Autodesk Fusion 360 part; units mm, degrees
note: some values were not read from the file. Set by a fixed rule: which sketch regions a step uses.
(part 36 of 59)
  spline S12 degree 5 poles (-26.8955, 1.5338) (-26.8956, 1.5338) (-26.8958, 1.5337) (-26.8961, 1.5336) (-26.8966, 1.5334) (-26.8973, 1.5331) (-26.8981, 1.5328) (-26.899, 1.5324) (-26.9, 1.5319) (-26.9011, 1.5315) (-26.9023, 1.5309) (-26.9036, 1.5304) (-26.905, 1.5298) (-26.9065, 1.5291) (-26.908, 1.5284) (-26.9097, 1.5276) (-26.9115, 1.5269) (-26.9134, 1.526) (-26.9153, 1.5251) (-26.9173, 1.5242) (-26.9195, 1.5232) (-26.9217, 1.5222) (-26.924, 1.5212) (-26.9263, 1.5201) (-26.9288, 1.5189) (-26.9313, 1.5177) (-26.9339, 1.5165) (-26.9366, 1.5152) (-26.9394, 1.5139) (-26.9423, 1.5125) (-26.9452, 1.5111) (-26.9482, 1.5097) (-26.9513, 1.5082) (-26.9544, 1.5066) (-26.9577, 1.5051) (-26.961, 1.5034) (-26.9643, 1.5018) (-26.9678, 1.5001) (-26.9713, 1.4983) (-26.9748, 1.4965) (-26.9785, 1.4947) (-26.9822, 1.4928) (-26.986, 1.4909) (-26.9898, 1.4889) (-26.9937, 1.4869) (-26.9977, 1.4849) (-27.0017, 1.4828) (-27.0058, 1.4807) (-27.01, 1.4785) (-27.0142, 1.4763) (-27.0185, 1.4741) (-27.0228, 1.4718) (-27.0272, 1.4694) (-27.0317, 1.4671) (-27.0362, 1.4647) (-27.0408, 1.4622) (-27.0454, 1.4597) (-27.0501, 1.4572) (-27.0549, 1.4546) (-27.0597, 1.452) (-27.0645, 1.4493) (-27.0694, 1.4466) (-27.0744, 1.4439) (-27.0794, 1.4411) (-27.0845, 1.4383) (-27.0896, 1.4354) (-27.0948, 1.4325) (-27.1, 1.4296) (-27.1053, 1.4266) (-27.1106, 1.4236) (-27.116, 1.4205) (-27.1214, 1.4174) (-27.1269, 1.4143) (-27.1324, 1.4111) (-27.138, 1.4079) (-27.1436, 1.4046) (-27.1493, 1.4013) (-27.155, 1.398) (-27.1608, 1.3946) (-27.1666, 1.3912) (-27.1725, 1.3877) (-27.1784, 1.3842) (-27.1843, 1.3807) (-27.1903, 1.3771) (-27.1963, 1.3735) (-27.2024, 1.3699) (-27.2085, 1.3662) (-27.2147, 1.3624) (-27.2209, 1.3587) (-27.2271, 1.3549) (-27.2334, 1.351) (-27.2397, 1.3471) (-27.2461, 1.3432) (-27.2525, 1.3392) (-27.259, 1.3352) (-27.2654, 1.3312) (-27.272, 1.3271) (-27.2785, 1.323) (-27.2851, 1.3188) (-27.2918, 1.3146) (-27.2985, 1.3104) (-27.3052, 1.3061) (-27.3119, 1.3018) (-27.3187, 1.2975) (-27.3256, 1.2931) (-27.3324, 1.2887) (-27.3393, 1.2842) (-27.3463, 1.2797) (-27.3533, 1.2752) (-27.3603, 1.2706) (-27.3673, 1.266) (-27.3744, 1.2613) (-27.3815, 1.2566) (-27.3887, 1.2519) (-27.3958, 1.2471) (-27.4031, 1.2423) (-27.4103, 1.2375) (-27.4176, 1.2326) (-27.4249, 1.2277) (-27.4323, 1.2227) (-27.4396, 1.2177) (-27.447, 1.2127) (-27.4545, 1.2076) (-27.462, 1.2025) (-27.4695, 1.1974) (-27.477, 1.1922) (-27.4846, 1.187) (-27.4922, 1.1817) (-27.4998, 1.1765) (-27.5074, 1.1711) (-27.5151, 1.1658) (-27.5228, 1.1604) (-27.5306, 1.1549) (-27.5384, 1.1494) (-27.5462, 1.1439) (-27.554, 1.1384) (-27.5618, 1.1328) (-27.5697, 1.1272) (-27.5776, 1.1215) (-27.5856, 1.1158) (-27.5936, 1.1101) (-27.6015, 1.1043) (-27.6096, 1.0985) (-27.6176, 1.0926) (-27.6257, 1.0868) (-27.6338, 1.0808) (-27.6419, 1.0749) (-27.6501, 1.0689) (-27.6582, 1.0629) (-27.6665, 1.0568) (-27.6747, 1.0507) (-27.6829, 1.0446) (-27.6912, 1.0384) (-27.6995, 1.0322) (-27.7078, 1.0259) (-27.7162, 1.0197) (-27.7246, 1.0133) (-27.733, 1.007) (-27.7414, 1.0006) (-27.7498, 0.9942) (-27.7583, 0.9877) (-27.7668, 0.9812) (-27.7753, 0.9747) (-27.7838, 0.9681) (-27.7924, 0.9615) (-27.801, 0.9548) (-27.8096, 0.9482) (-27.8182, 0.9415) (-27.8268, 0.9347) (-27.8355, 0.9279) (-27.8442, 0.9211) (-27.8529, 0.9142) (-27.8616, 0.9073) (-27.8704, 0.9004) (-27.8791, 0.8935) (-27.8879, 0.8865) (-27.8967, 0.8794) (-27.9055, 0.8724) (-27.9144, 0.8652) (-27.9233, 0.8581) (-27.9322, 0.8509) (-27.9411, 0.8437) (-27.95, 0.8365) (-27.9589, 0.8292) (-27.9679, 0.8219) (-27.9769, 0.8145) (-27.9859, 0.8071) (-27.9949, 0.7997) (-28.0039, 0.7922) (-28.013, 0.7847) (-28.0221, 0.7772) (-28.0312, 0.7697) (-28.0403, 0.7621) (-28.0494, 0.7544) (-28.0585, 0.7468) (-28.0677, 0.7391) (-28.0769, 0.7313) (-28.0861, 0.7235) (-28.0953, 0.7157) (-28.1045, 0.7079) (-28.1137, 0.7) (-28.123, 0.6921) (-28.1323, 0.6842) (-28.1416, 0.6762) (-28.1509, 0.6682) (-28.1602, 0.6601) (-28.1695, 0.652) (-28.1789, 0.6439) (-28.1882, 0.6357) (-28.1976, 0.6276) (-28.207, 0.6193) (-28.2164, 0.6111) (-28.2259, 0.6028) (-28.2353, 0.5945) (-28.2447, 0.5861) (-28.2542, 0.5777) (-28.2637, 0.5693) (-28.2732, 0.5608) (-28.2827, 0.5523) (-28.2922, 0.5438) (-28.3018, 0.5352) (-28.3113, 0.5266) (-28.3209, 0.518) (-28.3305, 0.5093) (-28.34, 0.5006) (-28.3496, 0.4919) (-28.3593, 0.4831) (-28.3689, 0.4743) (-28.3785, 0.4655) (-28.3882, 0.4566) (-28.3978, 0.4477) (-28.4075, 0.4387) (-28.4172, 0.4298) (-28.4269, 0.4208) (-28.4366, 0.4117) (-28.4464, 0.4027) (-28.4561, 0.3935) (-28.4658, 0.3844) (-28.4756, 0.3752) (-28.4854, 0.366) (-28.4951, 0.3568) (-28.503, 0.3494) (-28.5089, 0.3438) (-28.5128, 0.34) (-28.5147, 0.3382) knots 0 0 0 0 0 0 0.00416667 0.00833333 0.0125 0.01666667 0.02083333 0.025 0.02916667 0.03333333 0.0375 0.04166667 0.04583333 0.05 0.05416667 0.05833333 0.0625 0.06666667 0.07083333 0.075 0.07916667 0.08333333 0.0875 0.09166667 0.09583333 0.1 0.10416667 0.10833333 0.1125 0.11666667 0.12083333 0.125 0.12916667 0.13333333 0.1375 0.14166667 0.14583333 0.15 0.15416667 0.15833333 0.1625 0.16666667 0.17083333 0.175 0.17916667 0.18333333 0.1875 0.19166667 0.19583333 0.2 0.20416667 0.20833333 0.2125 0.21666667 0.22083333 0.225 0.22916667 0.23333333 0.2375 0.24166667 0.24583333 0.25 0.25416667 0.25833333 0.2625 0.26666667 0.27083333 0.275 0.27916667 0.28333333 0.2875 0.29166667 0.29583333 0.3 0.30416667 0.30833333 0.3125 0.31666667 0.32083333 0.325 0.32916667 0.33333333 0.3375 0.34166667 0.34583333 0.35 0.35416667 0.35833333 0.3625 0.36666667 0.37083333 0.375 0.37916667 0.38333333 0.3875 0.39166667 0.39583333 0.4 0.40416667 0.40833333 0.4125 0.41666667 0.42083333 0.425 0.42916667 0.43333333 0.4375 0.44166667 0.44583333 0.45 0.45416667 0.45833333 0.4625 0.46666667 0.47083333 0.475 0.47916667 0.48333333 0.4875 0.49166667 0.49583333 0.5 0.50416667 0.50833333 0.5125 0.51666667 0.52083333 0.525 0.52916667 0.53333333 0.5375 0.54166667 0.54583333 0.55 0.55416667 0.55833333 0.5625 0.56666667 0.57083333 0.575 0.57916667 0.58333333 0.5875 0.59166667 0.59583333 0.6 0.60416667 0.60833333 0.6125 0.61666667 0.62083333 0.625 0.62916667 0.63333333 0.6375 0.64166667 0.64583333 0.65 0.65416667 0.65833333 0.6625 0.66666667 0.67083333 0.675 0.67916667 0.68333333 0.6875 0.69166667 0.69583333 0.7 0.70416667 0.70833333 0.7125 0.71666667 0.72083333 0.725 0.72916667 0.73333333 0.7375 0.74166667 0.74583333 0.75 0.75416667 0.75833333 0.7625 0.76666667 0.77083333 0.775 0.77916667 0.78333333 0.7875 0.79166667 0.79583333 0.8 0.80416667 0.80833333 0.8125 0.81666667 0.82083333 0.825 0.82916667 0.83333333 0.8375 0.84166667 0.84583333 0.85 0.85416667 0.85833333 0.8625 0.86666667 0.87083333 0.875 0.87916667 0.88333333 0.8875 0.89166667 0.89583333 0.9 0.90416667 0.90833333 0.9125 0.91666667 0.92083333 0.925 0.92916667 0.93333333 0.9375 0.94166667 0.94583333 0.95 0.95416667 0.95833333 0.9625 0.96666667 0.97083333 0.975 0.97916667 0.98333333 0.9875 0.99166667 0.99583333 1 1 1 1 1 1
  arc A13 (-28.5147, 0.3382) -> (-28.1181, -0.5527) centre (0, 12.5) ccw
  spline S13 degree 5 poles (-28.1181, -0.5527) (-28.1154, -0.5525) (-28.11, -0.5521) (-28.1019, -0.5515) (-28.0911, -0.5506) (-28.0777, -0.5495) (-28.0644, -0.5484) (-28.051, -0.5473) (-28.0377, -0.5462) (-28.0244, -0.5451) (-28.0112, -0.5439) (-27.9979, -0.5427) (-27.9848, -0.5415) (-27.9716, -0.5404) (-27.9585, -0.5391) (-27.9454, -0.5379) (-27.9323, -0.5367) (-27.9193, -0.5354) (-27.9063, -0.5342) (-27.8934, -0.5329) (-27.8805, -0.5316) (-27.8676, -0.5303) (-27.8547, -0.529) (-27.8419, -0.5276) (-27.8291, -0.5263) (-27.8164, -0.5249) (-27.8037, -0.5236) (-27.791, -0.5222) (-27.7784, -0.5208) (-27.7658, -0.5194) (-27.7532, -0.518) (-27.7406, -0.5165) (-27.7281, -0.5151) (-27.7157, -0.5136) (-27.7032, -0.5122) (-27.6908, -0.5107) (-27.6785, -0.5092) (-27.6661, -0.5077) (-27.6539, -0.5062) (-27.6416, -0.5047) (-27.6294, -0.5031) (-27.6172, -0.5016) (-27.605, -0.5) (-27.5929, -0.4984) (-27.5809, -0.4968) (-27.5688, -0.4952) (-27.5568, -0.4936) (-27.5449, -0.492) (-27.5329, -0.4904) (-27.521, -0.4887) (-27.5092, -0.4871) (-27.4974, -0.4854) (-27.4856, -0.4838) (-27.4738, -0.4821) (-27.4621, -0.4804) (-27.4505, -0.4787) (-27.4388, -0.477) (-27.4273, -0.4752) (-27.4157, -0.4735) (-27.4042, -0.4718) (-27.3927, -0.47) (-27.3813, -0.4682) (-27.3699, -0.4665) (-27.3585, -0.4647) (-27.3472, -0.4629) (-27.3359, -0.4611) (-27.3247, -0.4593) (-27.3135, -0.4574) (-27.3023, -0.4556) (-27.2912, -0.4538) (-27.2801, -0.4519) (-27.2691, -0.4501) (-27.2581, -0.4482) (-27.2471, -0.4463) (-27.2362, -0.4445) (-27.2253, -0.4426) (-27.2145, -0.4407) (-27.2037, -0.4388) (-27.1929, -0.4368) (-27.1822, -0.4349) (-27.1715, -0.433) (-27.1609, -0.4311) (-27.1503, -0.4291) (-27.1397, -0.4272) (-27.1292, -0.4252) (-27.1188, -0.4232) (-27.1083, -0.4213) (-27.0979, -0.4193) (-27.0876, -0.4173) (-27.0773, -0.4153) (-27.0671, -0.4133) (-27.0568, -0.4113) (-27.0467, -0.4093) (-27.0365, -0.4072) (-27.0265, -0.4052) (-27.0164, -0.4032) (-27.0064, -0.4011) (-26.9965, -0.3991) (-26.9866, -0.3971) (-26.9767, -0.395) (-26.9669, -0.3929) (-26.9571, -0.3909) (-26.9474, -0.3888) (-26.9377, -0.3867) (-26.9281, -0.3847) (-26.9185, -0.3826) (-26.9089, -0.3805) (-26.8994, -0.3784) (-26.89, -0.3763) (-26.8806, -0.3742) (-26.8712, -0.3721) (-26.8619, -0.37) (-26.8526, -0.3679) (-26.8434, -0.3658) (-26.8342, -0.3636) (-26.8251, -0.3615) (-26.816, -0.3594) (-26.8069, -0.3573) (-26.798, -0.3551) (-26.789, -0.353) (-26.7801, -0.3509) (-26.7713, -0.3487) (-26.7625, -0.3466) (-26.7537, -0.3445) (-26.7451, -0.3423) (-26.7364, -0.3402) (-26.7278, -0.338) (-26.7193, -0.3359) (-26.7108, -0.3337) (-26.7023, -0.3316) (-26.6939, -0.3294) (-26.6856, -0.3273) (-26.6773, -0.3251) (-26.669, -0.323) (-26.6608, -0.3208) (-26.6527, -0.3187) (-26.6446, -0.3166) (-26.6365, -0.3144) (-26.6286, -0.3123) (-26.6206, -0.3101) (-26.6127, -0.308) (-26.6049, -0.3058) (-26.5971, -0.3037) (-26.5894, -0.3016) (-26.5817, -0.2994) (-26.5741, -0.2973) (-26.5665, -0.2952) (-26.559, -0.293) (-26.5516, -0.2909) (-26.5442, -0.2888) (-26.5368, -0.2867) (-26.5296, -0.2845) (-26.5223, -0.2824) (-26.5151, -0.2803) (-26.508, -0.2782) (-26.5009, -0.2761) (-26.4939, -0.274) (-26.487, -0.272) (-26.4801, -0.2699) (-26.4733, -0.2678) (-26.4665, -0.2657) (-26.4598, -0.2637) (-26.4531, -0.2616) (-26.4465, -0.2596) (-26.4399, -0.2575) (-26.4335, -0.2555) (-26.427, -0.2534) (-26.4207, -0.2514) (-26.4144, -0.2494) (-26.4081, -0.2474) (-26.4019, -0.2454) (-26.3958, -0.2434) (-26.3897, -0.2414) (-26.3837, -0.2395) (-26.3778, -0.2375) (-26.3719, -0.2356) (-26.3661, -0.2336) (-26.3604, -0.2317) (-26.3547, -0.2298) (-26.3491, -0.2279) (-26.3435, -0.226) (-26.338, -0.2241) (-26.3326, -0.2222) (-26.3273, -0.2204) (-26.322, -0.2185) (-26.3167, -0.2167) (-26.3116, -0.2149) (-26.3065, -0.2131) (-26.3015, -0.2113) (-26.2965, -0.2095) (-26.2916, -0.2077) (-26.2868, -0.206) (-26.282, -0.2043) (-26.2774, -0.2026) (-26.2728, -0.2009) (-26.2682, -0.1992) (-26.2638, -0.1975) (-26.2594, -0.1959) (-26.255, -0.1943) (-26.2508, -0.1927) (-26.2466, -0.1911) (-26.2425, -0.1895) (-26.2385, -0.188) (-26.2345, -0.1864) (-26.2307, -0.1849) (-26.2269, -0.1834) (-26.2231, -0.182) (-26.2195, -0.1806) (-26.2159, -0.1791) (-26.2124, -0.1778) (-26.209, -0.1764) (-26.2057, -0.175) (-26.2024, -0.1737) (-26.1993, -0.1724) (-26.1962, -0.1712) (-26.1932, -0.1699) (-26.1903, -0.1687) (-26.1874, -0.1676) (-26.1847, -0.1664) (-26.182, -0.1653) (-26.1794, -0.1642) (-26.1769, -0.1631) (-26.1745, -0.1621) (-26.1722, -0.1611) (-26.17, -0.1602) (-26.1678, -0.1592) (-26.1658, -0.1583) (-26.1638, -0.1575) (-26.1619, -0.1567) (-26.1602, -0.1559) (-26.1585, -0.1551) (-26.1569, -0.1544) (-26.1554, -0.1538) (-26.154, -0.1531) (-26.1527, -0.1526) (-26.1515, -0.152) (-26.1504, -0.1515) (-26.1495, -0.151) (-26.1486, -0.1506) (-26.1478, -0.1503) (-26.1471, -0.15) (-26.1467, -0.1497) (-26.1464, -0.1496) (-26.1462, -0.1495) (-26.1461, -0.1495) knots -1 -1 -1 -1 -1 -1 -0.99583333 -0.99166667 -0.9875 -0.98333333 -0.97916667 -0.975 -0.97083333 -0.96666667 -0.9625 -0.95833333 -0.95416667 -0.95 -0.94583333 -0.94166667 -0.9375 -0.93333333 -0.92916667 -0.925 -0.92083333 -0.91666667 -0.9125 -0.90833333 -0.90416667 -0.9 -0.89583333 -0.89166667 -0.8875 -0.88333333 -0.87916667 -0.875 -0.87083333 -0.86666667 -0.8625 -0.85833333 -0.85416667 -0.85 -0.84583333 -0.84166667 -0.8375 -0.83333333 -0.82916667 -0.825 -0.82083333 -0.81666667 -0.8125 -0.80833333 -0.80416667 -0.8 -0.79583333 -0.79166667 -0.7875 -0.78333333 -0.77916667 -0.775 -0.77083333 -0.76666667 -0.7625 -0.75833333 -0.75416667 -0.75 -0.74583333 -0.74166667 -0.7375 -0.73333333 -0.72916667 -0.725 -0.72083333 -0.71666667 -0.7125 -0.70833333 -0.70416667 -0.7 -0.69583333 -0.69166667 -0.6875 -0.68333333 -0.67916667 -0.675 -0.67083333 -0.66666667 -0.6625 -0.65833333 -0.65416667 -0.65 -0.64583333 -0.64166667 -0.6375 -0.63333333 -0.62916667 -0.625 -0.62083333 -0.61666667 -0.6125 -0.60833333 -0.60416667 -0.6 -0.59583333 -0.59166667 -0.5875 -0.58333333 -0.57916667 -0.575 -0.57083333 -0.56666667 -0.5625 -0.55833333 -0.55416667 -0.55 -0.54583333 -0.54166667 -0.5375 -0.53333333 -0.52916667 -0.525 -0.52083333 -0.51666667 -0.5125 -0.50833333 -0.50416667 -0.5 -0.49583333 -0.49166667 -0.4875 -0.48333333 -0.47916667 -0.475 -0.47083333 -0.46666667 -0.4625 -0.45833333 -0.45416667 -0.45 -0.44583333 -0.44166667 -0.4375 -0.43333333 -0.42916667 -0.425 -0.42083333 -0.41666667 -0.4125 -0.40833333 -0.40416667 -0.4 -0.39583333 -0.39166667 -0.3875 -0.38333333 -0.37916667 -0.375 -0.37083333 -0.36666667 -0.3625 -0.35833333 -0.35416667 -0.35 -0.34583333 -0.34166667 -0.3375 -0.33333333 -0.32916667 -0.325 -0.32083333 -0.31666667 -0.3125 -0.30833333 -0.30416667 -0.3 -0.29583333 -0.29166667 -0.2875 -0.28333333 -0.27916667 -0.275 -0.27083333 -0.26666667 -0.2625 -0.25833333 -0.25416667 -0.25 -0.24583333 -0.24166667 -0.2375 -0.23333333 -0.22916667 -0.225 -0.22083333 -0.21666667 -0.2125 -0.20833333 -0.20416667 -0.2 -0.19583333 -0.19166667 -0.1875 -0.18333333 -0.17916667 -0.175 -0.17083333 -0.16666667 -0.1625 -0.15833333 -0.15416667 -0.15 -0.14583333 -0.14166667 -0.1375 -0.13333333 -0.12916667 -0.125 -0.12083333 -0.11666667 -0.1125 -0.10833333 -0.10416667 -0.1 -0.09583333 -0.09166667 -0.0875 -0.08333333 -0.07916667 -0.075 -0.07083333 -0.06666667 -0.0625 -0.05833333 -0.05416667 -0.05 -0.04583333 -0.04166667 -0.0375 -0.03333333 -0.02916667 -0.025 -0.02083333 -0.01666667 -0.0125 -0.00833333 -0.00416667 0 0 0 0 0 0
  line L35 (-26.1461, -0.1495) -> (-26.1453, -0.1491)
  line L36 (-26.1453, -0.1491) -> (-25.8803, -0.0209)
  arc A14 (-25.8803, -0.0209) -> (-25.3417, -1.078) centre (0, 12.5) ccw
  line L37 (-25.3417, -1.078) -> (-25.6012, -1.2171)
  line L38 (-25.6012, -1.2171) -> (-25.6019, -1.2175)
  spline S14 degree 5 poles (-25.6019, -1.2175) (-25.602, -1.2175) (-25.6022, -1.2176) (-25.6025, -1.2178) (-25.6029, -1.218) (-25.6036, -1.2184) (-25.6043, -1.2188) (-25.6052, -1.2193) (-25.6061, -1.2198) (-25.6072, -1.2204) (-25.6083, -1.221) (-25.6096, -1.2217) (-25.6109, -1.2225) (-25.6123, -1.2233) (-25.6138, -1.2242) (-25.6154, -1.2251) (-25.6171, -1.2261) (-25.6188, -1.2271) (-25.6207, -1.2282) (-25.6226, -1.2293) (-25.6246, -1.2305) (-25.6267, -1.2317) (-25.6289, -1.233) (-25.6311, -1.2344) (-25.6334, -1.2358) (-25.6358, -1.2372) (-25.6383, -1.2387) (-25.6409, -1.2403) (-25.6435, -1.2419) (-25.6462, -1.2435) (-25.6489, -1.2452) (-25.6518, -1.247) (-25.6547, -1.2488) (-25.6577, -1.2506) (-25.6607, -1.2526) (-25.6638, -1.2545) (-25.667, -1.2565) (-25.6702, -1.2586) (-25.6735, -1.2607) (-25.6769, -1.2628) (-25.6803, -1.265) (-25.6838, -1.2673) (-25.6874, -1.2696) (-25.691, -1.2719) (-25.6947, -1.2743) (-25.6984, -1.2768) (-25.7022, -1.2793) (-25.706, -1.2818) (-25.71, -1.2844) (-25.7139, -1.287) (-25.718, -1.2897) (-25.722, -1.2925) (-25.7262, -1.2952) (-25.7304, -1.2981) (-25.7346, -1.3009) (-25.7389, -1.3039) (-25.7432, -1.3068) (-25.7476, -1.3098) (-25.7521, -1.3129) (-25.7566, -1.316) (-25.7612, -1.3192) (-25.7658, -1.3224) (-25.7704, -1.3256) (-25.7751, -1.3289) (-25.7799, -1.3322) (-25.7847, -1.3356) (-25.7895, -1.339) (-25.7944, -1.3425) (-25.7993, -1.346) (-25.8043, -1.3496) (-25.8093, -1.3532) (-25.8144, -1.3568) (-25.8195, -1.3605) (-25.8247, -1.3643) (-25.8299, -1.3681) (-25.8352, -1.3719) (-25.8405, -1.3758) (-25.8458, -1.3797) (-25.8512, -1.3836) (-25.8566, -1.3876) (-25.8621, -1.3917) (-25.8676, -1.3958) (-25.8731, -1.3999) (-25.8787, -1.4041) (-25.8843, -1.4083) (-25.89, -1.4126) (-25.8957, -1.4169) (-25.9014, -1.4213) (-25.9072, -1.4257) (-25.913, -1.4301) (-25.9188, -1.4346) (-25.9247, -1.4391) (-25.9306, -1.4437) (-25.9366, -1.4483) (-25.9426, -1.4529) (-25.9486, -1.4576) (-25.9547, -1.4624) (-25.9608, -1.4672) (-25.9669, -1.472) (-25.9731, -1.4769) (-25.9793, -1.4818) (-25.9855, -1.4867) (-25.9918, -1.4917) (-25.9981, -1.4967) (-26.0044, -1.5018) (-26.0108, -1.5069) (-26.0172, -1.5121) (-26.0236, -1.5173) (-26.0301, -1.5225) (-26.0366, -1.5278) (-26.0431, -1.5332) (-26.0497, -1.5385) (-26.0563, -1.5439) (-26.0629, -1.5494) (-26.0695, -1.5549) (-26.0762, -1.5604) (-26.0829, -1.566) (-26.0896, -1.5716) (-26.0964, -1.5772) (-26.1032, -1.5829) (-26.11, -1.5887) (-26.1168, -1.5945) (-26.1237, -1.6003) (-26.1306, -1.6061) (-26.1375, -1.612) (-26.1445, -1.618) (-26.1515, -1.6239) (-26.1585, -1.63) (-26.1655, -1.636) (-26.1726, -1.6421) (-26.1796, -1.6483) (-26.1868, -1.6544) (-26.1939, -1.6607) (-26.201, -1.6669) (-26.2082, -1.6732) (-26.2154, -1.6796) (-26.2227, -1.6859) (-26.2299, -1.6924) (-26.2372, -1.6988) (-26.2445, -1.7053) (-26.2518, -1.7119) (-26.2592, -1.7184) (-26.2665, -1.725) (-26.2739, -1.7317) (-26.2813, -1.7384) (-26.2888, -1.7451) (-26.2962, -1.7519) (-26.3037, -1.7587) (-26.3112, -1.7656) (-26.3188, -1.7724) (-26.3263, -1.7794) (-26.3339, -1.7863) (-26.3414, -1.7933) (-26.3491, -1.8004) (-26.3567, -1.8075) (-26.3643, -1.8146) (-26.372, -1.8217) (-26.3797, -1.8289) (-26.3874, -1.8362) (-26.3951, -1.8435) (-26.4029, -1.8508) (-26.4106, -1.8581) (-26.4184, -1.8655) (-26.4262, -1.8729) (-26.434, -1.8804) (-26.4419, -1.8879) (-26.4497, -1.8954) (-26.4576, -1.903) (-26.4655, -1.9106) (-26.4734, -1.9183) (-26.4813, -1.926) (-26.4893, -1.9337) (-26.4972, -1.9415) (-26.5052, -1.9493) (-26.5132, -1.9571) (-26.5212, -1.965) (-26.5292, -1.9729) (-26.5373, -1.9809) (-26.5453, -1.9889) (-26.5534, -1.9969) (-26.5615, -2.005) (-26.5696, -2.0131) (-26.5777, -2.0212) (-26.5858, -2.0294) (-26.594, -2.0376) (-26.6022, -2.0459) (-26.6103, -2.0541) (-26.6185, -2.0625) (-26.6267, -2.0708) (-26.635, -2.0792) (-26.6432, -2.0877) (-26.6514, -2.0961) (-26.6597, -2.1046) (-26.668, -2.1132) (-26.6763, -2.1218) (-26.6846, -2.1304) (-26.6929, -2.139) (-26.7012, -2.1477) (-26.7096, -2.1565) (-26.7179, -2.1652) (-26.7263, -2.174) (-26.7347, -2.1829) (-26.7431, -2.1917) (-26.7515, -2.2006) (-26.7599, -2.2096) (-26.7683, -2.2186) (-26.7767, -2.2276) (-26.7852, -2.2366) (-26.7937, -2.2457) (-26.8021, -2.2549) (-26.8106, -2.264) (-26.8191, -2.2732) (-26.8276, -2.2824) (-26.8361, -2.2917) (-26.8447, -2.301) (-26.8532, -2.3104) (-26.8618, -2.3197) (-26.8703, -2.3291) (-26.8789, -2.3386) (-26.8875, -2.3481) (-26.8961, -2.3576) (-26.9047, -2.3671) (-26.9133, -2.3767) (-26.9219, -2.3863) (-26.9305, -2.396) (-26.9392, -2.4057) (-26.9478, -2.4154) (-26.9565, -2.4252) (-26.9651, -2.435) (-26.9738, -2.4448) (-26.9825, -2.4547) (-26.9912, -2.4646) (-26.9999, -2.4745) (-27.0086, -2.4845) (-27.0173, -2.4945) (-27.026, -2.5045) (-27.0347, -2.5146) (-27.0435, -2.5247) (-27.0522, -2.5349) (-27.061, -2.545) (-27.0697, -2.5553) (-27.0767, -2.5635) (-27.082, -2.5696) (-27.0855, -2.5737) (-27.0873, -2.5758) knots 0 0 0 0 0 0 0.00416667 0.00833333 0.0125 0.01666667 0.02083333 0.025 0.02916667 0.03333333 0.0375 0.04166667 0.04583333 0.05 0.05416667 0.05833333 0.0625 0.06666667 0.07083333 0.075 0.07916667 0.08333333 0.0875 0.09166667 0.09583333 0.1 0.10416667 0.10833333 0.1125 0.11666667 0.12083333 0.125 0.12916667 0.13333333 0.1375 0.14166667 0.14583333 0.15 0.15416667 0.15833333 0.1625 0.16666667 0.17083333 0.175 0.17916667 0.18333333 0.1875 0.19166667 0.19583333 0.2 0.20416667 0.20833333 0.2125 0.21666667 0.22083333 0.225 0.22916667 0.23333333 0.2375 0.24166667 0.24583333 0.25 0.25416667 0.25833333 0.2625 0.26666667 0.27083333 0.275 0.27916667 0.28333333 0.2875 0.29166667 0.29583333 0.3 0.30416667 0.30833333 0.3125 0.31666667 0.32083333 0.325 0.32916667 0.33333333 0.3375 0.34166667 0.34583333 0.35 0.35416667 0.35833333 0.3625 0.36666667 0.37083333 0.375 0.37916667 0.38333333 0.3875 0.39166667 0.39583333 0.4 0.40416667 0.40833333 0.4125 0.41666667 0.42083333 0.425 0.42916667 0.43333333 0.4375 0.44166667 0.44583333 0.45 0.45416667 0.45833333 0.4625 0.46666667 0.47083333 0.475 0.47916667 0.48333333 0.4875 0.49166667 0.49583333 0.5 0.50416667 0.50833333 0.5125 0.51666667 0.52083333 0.525 0.52916667 0.53333333 0.5375 0.54166667 0.54583333 0.55 0.55416667 0.55833333 0.5625 0.56666667 0.57083333 0.575 0.57916667 0.58333333 0.5875 0.59166667 0.59583333 0.6 0.60416667 0.60833333 0.6125 0.61666667 0.62083333 0.625 0.62916667 0.63333333 0.6375 0.64166667 0.64583333 0.65 0.65416667 0.65833333 0.6625 0.66666667 0.67083333 0.675 0.67916667 0.68333333 0.6875 0.69166667 0.69583333 0.7 0.70416667 0.70833333 0.7125 0.71666667 0.72083333 0.725 0.72916667 0.73333333 0.7375 0.74166667 0.74583333 0.75 0.75416667 0.75833333 0.7625 0.76666667 0.77083333 0.775 0.77916667 0.78333333 0.7875 0.79166667 0.79583333 0.8 0.80416667 0.80833333 0.8125 0.81666667 0.82083333 0.825 0.82916667 0.83333333 0.8375 0.84166667 0.84583333 0.85 0.85416667 0.85833333 0.8625 0.86666667 0.87083333 0.875 0.87916667 0.88333333 0.8875 0.89166667 0.89583333 0.9 0.90416667 0.90833333 0.9125 0.91666667 0.92083333 0.925 0.92916667 0.93333333 0.9375 0.94166667 0.94583333 0.95 0.95416667 0.95833333 0.9625 0.96666667 0.97083333 0.975 0.97916667 0.98333333 0.9875 0.99166667 0.99583333 1 1 1 1 1 1
  arc A15 (-27.0873, -2.5758) -> (-26.5997, -3.4204) centre (0, 12.5) ccw
  spline S15 degree 5 poles (-26.5997, -3.4204) (-26.597, -3.4199) (-26.5917, -3.4189) (-26.5837, -3.4174) (-26.5731, -3.4154) (-26.5599, -3.413) (-26.5467, -3.4105) (-26.5335, -3.408) (-26.5204, -3.4055) (-26.5073, -3.4029) (-26.4943, -3.4004) (-26.4812, -3.3979) (-26.4682, -3.3953) (-26.4553, -3.3927) (-26.4424, -3.3902) (-26.4295, -3.3876) (-26.4166, -3.385) (-26.4038, -3.3824) (-26.391, -3.3798) (-26.3783, -3.3771) (-26.3656, -3.3745) (-26.3529, -3.3719) (-26.3403, -3.3692) (-26.3276, -3.3666) (-26.3151, -3.3639) (-26.3025, -3.3612) (-26.29, -3.3585) (-26.2776, -3.3558) (-26.2651, -3.3531) (-26.2528, -3.3504) (-26.2404, -3.3477) (-26.2281, -3.3449) (-26.2158, -3.3422) (-26.2035, -3.3394) (-26.1913, -3.3367) (-26.1792, -3.3339) (-26.167, -3.3311) (-26.1549, -3.3283) (-26.1428, -3.3255) (-26.1308, -3.3227) (-26.1188, -3.3199) (-26.1069, -3.3171) (-26.095, -3.3143) (-26.0831, -3.3115) (-26.0712, -3.3086) (-26.0594, -3.3058) (-26.0477, -3.3029) (-26.0359, -3.3001) (-26.0242, -3.2972) (-26.0126, -3.2943) (-26.001, -3.2914) (-25.9894, -3.2886) (-25.9778, -3.2857) (-25.9663, -3.2828) (-25.9549, -3.2798) (-25.9435, -3.2769) (-25.9321, -3.274) (-25.9207, -3.2711) (-25.9094, -3.2682) (-25.8982, -3.2652) (-25.8869, -3.2623) (-25.8757, -3.2593) (-25.8646, -3.2564) (-25.8535, -3.2534) (-25.8424, -3.2504) (-25.8314, -3.2475) (-25.8204, -3.2445) (-25.8094, -3.2415) (-25.7985, -3.2385) (-25.7877, -3.2355) (-25.7768, -3.2325) (-25.766, -3.2295) (-25.7553, -3.2265) (-25.7446, -3.2235) (-25.7339, -3.2205) (-25.7233, -3.2175) (-25.7127, -3.2145) (-25.7022, -3.2114) (-25.6917, -3.2084) (-25.6812, -3.2054) (-25.6708, -3.2023) (-25.6604, -3.1993) (-25.6501, -3.1963) (-25.6398, -3.1932) (-25.6296, -3.1902) (-25.6194, -3.1871) (-25.6092, -3.1841) (-25.5991, -3.181) (-25.589, -3.1779) (-25.579, -3.1749) (-25.569, -3.1718) (-25.559, -3.1688) (-25.5491, -3.1657) (-25.5393, -3.1626) (-25.5294, -3.1596) (-25.5197, -3.1565) (-25.5099, -3.1534) (-25.5003, -3.1503) (-25.4906, -3.1473) (-25.481, -3.1442) (-25.4715, -3.1411) (-25.462, -3.138) (-25.4525, -3.135) (-25.4431, -3.1319) (-25.4337, -3.1288) (-25.4244, -3.1257) (-25.4151, -3.1227) (-25.4059, -3.1196) (-25.3967, -3.1165) (-25.3876, -3.1134) (-25.3785, -3.1104) (-25.3694, -3.1073) (-25.3604, -3.1042) (-25.3515, -3.1012) (-25.3426, -3.0981) (-25.3337, -3.095) (-25.3249, -3.092) (-25.3161, -3.0889) (-25.3074, -3.0859) (-25.2988, -3.0828) (-25.2901, -3.0798) (-25.2816, -3.0767) (-25.2731, -3.0737) (-25.2646, -3.0706) (-25.2562, -3.0676) (-25.2478, -3.0645) (-25.2394, -3.0615) (-25.2312, -3.0585) (-25.2229, -3.0555) (-25.2148, -3.0524) (-25.2066, -3.0494) (-25.1986, -3.0464) (-25.1905, -3.0434) (-25.1826, -3.0404) (-25.1746, -3.0374) (-25.1668, -3.0344) (-25.1589, -3.0315) (-25.1512, -3.0285) (-25.1434, -3.0255) (-25.1358, -3.0226) (-25.1282, -3.0196) (-25.1206, -3.0166) (-25.1131, -3.0137) (-25.1056, -3.0108) (-25.0982, -3.0078) (-25.0909, -3.0049) (-25.0836, -3.002) (-25.0763, -2.9991) (-25.0691, -2.9962) (-25.062, -2.9933) (-25.0549, -2.9905) (-25.0479, -2.9876) (-25.0409, -2.9848) (-25.034, -2.9819) (-25.0271, -2.9791) (-25.0203, -2.9762) (-25.0136, -2.9734) (-25.0069, -2.9706) (-25.0002, -2.9678) (-24.9936, -2.9651) (-24.9871, -2.9623) (-24.9806, -2.9595) (-24.9742, -2.9568) (-24.9679, -2.9541) (-24.9616, -2.9514) (-24.9553, -2.9486) (-24.9492, -2.946) (-24.943, -2.9433) (-24.937, -2.9406) (-24.931, -2.938) (-24.925, -2.9353) (-24.9192, -2.9327) (-24.9133, -2.9301) (-24.9076, -2.9275) (-24.9019, -2.925) (-24.8962, -2.9224) (-24.8907, -2.9199) (-24.8852, -2.9174) (-24.8797, -2.9149) (-24.8743, -2.9124) (-24.869, -2.9099) (-24.8637, -2.9075) (-24.8585, -2.905) (-24.8534, -2.9026) (-24.8483, -2.9002) (-24.8433, -2.8979) (-24.8384, -2.8955) (-24.8335, -2.8932) (-24.8287, -2.8909) (-24.8239, -2.8886) (-24.8193, -2.8863) (-24.8147, -2.8841) (-24.8101, -2.8819) (-24.8056, -2.8797) (-24.8012, -2.8775) (-24.7969, -2.8754) (-24.7926, -2.8733) (-24.7884, -2.8712) (-24.7843, -2.8691) (-24.7802, -2.8671) (-24.7763, -2.8651) (-24.7723, -2.8631) (-24.7685, -2.8611) (-24.7647, -2.8592) (-24.761, -2.8573) (-24.7574, -2.8554) (-24.7539, -2.8536) (-24.7504, -2.8518) (-24.747, -2.85) (-24.7437, -2.8482) (-24.7404, -2.8465) (-24.7372, -2.8449) (-24.7341, -2.8432) (-24.7311, -2.8416) (-24.7282, -2.84) (-24.7253, -2.8385) (-24.7225, -2.837) (-24.7198, -2.8355) (-24.7172, -2.8341) (-24.7147, -2.8327) (-24.7122, -2.8313) (-24.7099, -2.83) (-24.7076, -2.8287) (-24.7054, -2.8275) (-24.7033, -2.8263) (-24.7012, -2.8252) (-24.6993, -2.8241) (-24.6974, -2.823) (-24.6956, -2.822) (-24.694, -2.821) (-24.6924, -2.8201) (-24.6909, -2.8193) (-24.6895, -2.8184) (-24.6881, -2.8177) (-24.6869, -2.8169) (-24.6858, -2.8163) (-24.6848, -2.8157) (-24.6838, -2.8151) (-24.683, -2.8146) (-24.6822, -2.8142) (-24.6816, -2.8138) (-24.6812, -2.8135) (-24.6809, -2.8133) (-24.6807, -2.8132) (-24.6806, -2.8132) knots -1 -1 -1 -1 -1 -1 -0.99583333 -0.99166667 -0.9875 -0.98333333 -0.97916667 -0.975 -0.97083333 -0.96666667 -0.9625 -0.95833333 -0.95416667 -0.95 -0.94583333 -0.94166667 -0.9375 -0.93333333 -0.92916667 -0.925 -0.92083333 -0.91666667 -0.9125 -0.90833333 -0.90416667 -0.9 -0.89583333 -0.89166667 -0.8875 -0.88333333 -0.87916667 -0.875 -0.87083333 -0.86666667 -0.8625 -0.85833333 -0.85416667 -0.85 -0.84583333 -0.84166667 -0.8375 -0.83333333 -0.82916667 -0.825 -0.82083333 -0.81666667 -0.8125 -0.80833333 -0.80416667 -0.8 -0.79583333 -0.79166667 -0.7875 -0.78333333 -0.77916667 -0.775 -0.77083333 -0.76666667 -0.7625 -0.75833333 -0.75416667 -0.75 -0.74583333 -0.74166667 -0.7375 -0.73333333 -0.72916667 -0.725 -0.72083333 -0.71666667 -0.7125 -0.70833333 -0.70416667 -0.7 -0.69583333 -0.69166667 -0.6875 -0.68333333 -0.67916667 -0.675 -0.67083333 -0.66666667 -0.6625 -0.65833333 -0.65416667 -0.65 -0.64583333 -0.64166667 -0.6375 -0.63333333 -0.62916667 -0.625 -0.62083333 -0.61666667 -0.6125 -0.60833333 -0.60416667 -0.6 -0.59583333 -0.59166667 -0.5875 -0.58333333 -0.57916667 -0.575 -0.57083333 -0.56666667 -0.5625 -0.55833333 -0.55416667 -0.55 -0.54583333 -0.54166667 -0.5375 -0.53333333 -0.52916667 -0.525 -0.52083333 -0.51666667 -0.5125 -0.50833333 -0.50416667 -0.5 -0.49583333 -0.49166667 -0.4875 -0.48333333 -0.47916667 -0.475 -0.47083333 -0.46666667 -0.4625 -0.45833333 -0.45416667 -0.45 -0.44583333 -0.44166667 -0.4375 -0.43333333 -0.42916667 -0.425 -0.42083333 -0.41666667 -0.4125 -0.40833333 -0.40416667 -0.4 -0.39583333 -0.39166667 -0.3875 -0.38333333 -0.37916667 -0.375 -0.37083333 -0.36666667 -0.3625 -0.35833333 -0.35416667 -0.35 -0.34583333 -0.34166667 -0.3375 -0.33333333 -0.32916667 -0.325 -0.32083333 -0.31666667 -0.3125 -0.30833333 -0.30416667 -0.3 -0.29583333 -0.29166667 -0.2875 -0.28333333 -0.27916667 -0.275 -0.27083333 -0.26666667 -0.2625 -0.25833333 -0.25416667 -0.25 -0.24583333 -0.24166667 -0.2375 -0.23333333 -0.22916667 -0.225 -0.22083333 -0.21666667 -0.2125 -0.20833333 -0.20416667 -0.2 -0.19583333 -0.19166667 -0.1875 -0.18333333 -0.17916667 -0.175 -0.17083333 -0.16666667 -0.1625 -0.15833333 -0.15416667 -0.15 -0.14583333 -0.14166667 -0.1375 -0.13333333 -0.12916667 -0.125 -0.12083333 -0.11666667 -0.1125 -0.10833333 -0.10416667 -0.1 -0.09583333 -0.09166667 -0.0875 -0.08333333 -0.07916667 -0.075 -0.07083333 -0.06666667 -0.0625 -0.05833333 -0.05416667 -0.05 -0.04583333 -0.04166667 -0.0375 -0.03333333 -0.02916667 -0.025 -0.02083333 -0.01666667 -0.0125 -0.00833333 -0.00416667 0 0 0 0 0 0
  line L39 (-24.6806, -2.8132) -> (-24.6799, -2.8128)
  line L40 (-24.6799, -2.8128) -> (-24.4297, -2.6575)
  arc A16 (-24.4297, -2.6575) -> (-23.7836, -3.6526) centre (0, 12.5) ccw
  line L41 (-23.7836, -3.6526) -> (-24.0271, -3.818)
  line L42 (-24.0271, -3.818) -> (-24.0278, -3.8184)
  spline S16 degree 5 poles (-24.0278, -3.8184) (-24.0279, -3.8185) (-24.0281, -3.8186) (-24.0283, -3.8188) (-24.0287, -3.8191) (-24.0294, -3.8195) (-24.0301, -3.82) (-24.0309, -3.8206) (-24.0317, -3.8212) (-24.0327, -3.8219) (-24.0338, -3.8227) (-24.035, -3.8235) (-24.0362, -3.8244) (-24.0375, -3.8253) (-24.0389, -3.8263) (-24.0404, -3.8274) (-24.042, -3.8286) (-24.0436, -3.8298) (-24.0453, -3.831) (-24.0471, -3.8324) (-24.049, -3.8338) (-24.051, -3.8352) (-24.053, -3.8367) (-24.0551, -3.8383) (-24.0572, -3.8399) (-24.0595, -3.8416) (-24.0618, -3.8434) (-24.0641, -3.8452) (-24.0666, -3.8471) (-24.0691, -3.849) (-24.0717, -3.851) (-24.0743, -3.853) (-24.077, -3.8551) (-24.0798, -3.8573) (-24.0826, -3.8595) (-24.0855, -3.8618) (-24.0884, -3.8641) (-24.0914, -3.8665) (-24.0945, -3.8689) (-24.0976, -3.8714) (-24.1008, -3.874) (-24.104, -3.8766) (-24.1073, -3.8792) (-24.1107, -3.8819) (-24.1141, -3.8847) (-24.1176, -3.8875) (-24.1211, -3.8904) (-24.1246, -3.8933) (-24.1283, -3.8963) (-24.1319, -3.8994) (-24.1356, -3.9024) (-24.1394, -3.9056) (-24.1432, -3.9088) (-24.1471, -3.912) (-24.151, -3.9153) (-24.155, -3.9187) (-24.159, -3.9221) (-24.1631, -3.9256) (-24.1672, -3.9291) (-24.1713, -3.9326) (-24.1755, -3.9362) (-24.1798, -3.9399) (-24.1841, -3.9436) (-24.1884, -3.9474) (-24.1928, -3.9512) (-24.1972, -3.955) (-24.2017, -3.959) (-24.2062, -3.9629) (-24.2107, -3.9669) (-24.2153, -3.971) (-24.2199, -3.9751) (-24.2246, -3.9793) (-24.2293, -3.9835) (-24.234, -3.9877) (-24.2388, -3.992) (-24.2436, -3.9964) (-24.2485, -4.0008) (-24.2534, -4.0053) (-24.2583, -4.0098) (-24.2633, -4.0143) (-24.2683, -4.0189) (-24.2733, -4.0236) (-24.2784, -4.0282) (-24.2835, -4.033) (-24.2887, -4.0378) (-24.2939, -4.0426) (-24.2991, -4.0475) (-24.3043, -4.0524) (-24.3096, -4.0574) (-24.3149, -4.0624) (-24.3203, -4.0675) (-24.3257, -4.0726) (-24.3311, -4.0778) (-24.3365, -4.083) (-24.342, -4.0882) (-24.3475, -4.0935) (-24.353, -4.0989) (-24.3586, -4.1043) (-24.3642, -4.1097) (-24.3698, -4.1152) (-24.3755, -4.1207) (-24.3812, -4.1263) (-24.3869, -4.1319) (-24.3926, -4.1376) (-24.3984, -4.1433) (-24.4042, -4.1491) (-24.41, -4.1549) (-24.4159, -4.1607) (-24.4218, -4.1666) (-24.4277, -4.1725) (-24.4336, -4.1785) (-24.4395, -4.1845) (-24.4455, -4.1906) (-24.4515, -4.1967) (-24.4576, -4.2029) (-24.4636, -4.2091) (-24.4697, -4.2153) (-24.4758, -4.2216) (-24.482, -4.2279) (-24.4881, -4.2343) (-24.4943, -4.2407) (-24.5005, -4.2472) (-24.5067, -4.2537) (-24.513, -4.2602) (-24.5192, -4.2668) (-24.5255, -4.2735) (-24.5319, -4.2801) (-24.5382, -4.2869) (-24.5446, -4.2936) (-24.5509, -4.3004) (-24.5573, -4.3073) (-24.5638, -4.3142) (-24.5702, -4.3211) (-24.5767, -4.3281) (-24.5831, -4.3351) (-24.5897, -4.3421) (-24.5962, -4.3492) (-24.6027, -4.3564) (-24.6093, -4.3636) (-24.6159, -4.3708) (-24.6225, -4.3781) (-24.6291, -4.3854) (-24.6357, -4.3927) (-24.6424, -4.4001) (-24.6491, -4.4075) (-24.6558, -4.415) (-24.6625, -4.4225) (-24.6692, -4.4301) (-24.6759, -4.4377) (-24.6827, -4.4453) (-24.6895, -4.453) (-24.6963, -4.4607) (-24.7031, -4.4685) (-24.7099, -4.4763) (-24.7168, -4.4841) (-24.7236, -4.492) (-24.7305, -4.4999) (-24.7374, -4.5079) (-24.7443, -4.5159) (-24.7512, -4.5239) (-24.7582, -4.532) (-24.7651, -4.5401) (-24.7721, -4.5483) (-24.7791, -4.5565) (-24.7861, -4.5647) (-24.7931, -4.573) (-24.8001, -4.5813) (-24.8071, -4.5897) (-24.8142, -4.5981) (-24.8212, -4.6065) (-24.8283, -4.615) (-24.8354, -4.6235) (-24.8425, -4.6321) (-24.8496, -4.6407) (-24.8568, -4.6493) (-24.8639, -4.658) (-24.8711, -4.6667) (-24.8782, -4.6754) (-24.8854, -4.6842) (-24.8926, -4.6931) (-24.8998, -4.7019) (-24.907, -4.7108) (-24.9142, -4.7198) (-24.9215, -4.7288) (-24.9287, -4.7378) (-24.936, -4.7469) (-24.9432, -4.7559) (-24.9505, -4.7651) (-24.9578, -4.7743) (-24.9651, -4.7835) (-24.9724, -4.7927) (-24.9797, -4.802) (-24.9871, -4.8113) (-24.9944, -4.8207) (-25.0017, -4.8301) (-25.0091, -4.8395) (-25.0165, -4.849) (-25.0238, -4.8585) (-25.0312, -4.8681) (-25.0386, -4.8777) (-25.046, -4.8873) (-25.0534, -4.897) (-25.0609, -4.9067) (-25.0683, -4.9164) (-25.0757, -4.9262) (-25.0832, -4.936) (-25.0906, -4.9458) (-25.0981, -4.9557) (-25.1055, -4.9657) (-25.113, -4.9756) (-25.1205, -4.9856) (-25.128, -4.9956) (-25.1355, -5.0057) (-25.143, -5.0158) (-25.1505, -5.026) (-25.158, -5.0361) (-25.1655, -5.0464) (-25.1731, -5.0566) (-25.1806, -5.0669) (-25.1881, -5.0772) (-25.1957, -5.0876) (-25.2032, -5.098) (-25.2108, -5.1084) (-25.2184, -5.1189) (-25.2259, -5.1294) (-25.2335, -5.1399) (-25.2411, -5.1505) (-25.2487, -5.1611) (-25.2563, -5.1718) (-25.2639, -5.1825) (-25.2715, -5.1932) (-25.2791, -5.2039) (-25.2867, -5.2147) (-25.2943, -5.2256) (-25.3019, -5.2364) (-25.3096, -5.2473) (-25.3172, -5.2583) (-25.3248, -5.2692) (-25.3325, -5.2802) (-25.3401, -5.2913) (-25.3477, -5.3023) (-25.3539, -5.3112) (-25.3584, -5.3179) (-25.3615, -5.3224) (-25.363, -5.3246) knots 0 0 0 0 0 0 0.00416667 0.00833333 0.0125 0.01666667 0.02083333 0.025 0.02916667 0.03333333 0.0375 0.04166667 0.04583333 0.05 0.05416667 0.05833333 0.0625 0.06666667 0.07083333 0.075 0.07916667 0.08333333 0.0875 0.09166667 0.09583333 0.1 0.10416667 0.10833333 0.1125 0.11666667 0.12083333 0.125 0.12916667 0.13333333 0.1375 0.14166667 0.14583333 0.15 0.15416667 0.15833333 0.1625 0.16666667 0.17083333 0.175 0.17916667 0.18333333 0.1875 0.19166667 0.19583333 0.2 0.20416667 0.20833333 0.2125 0.21666667 0.22083333 0.225 0.22916667 0.23333333 0.2375 0.24166667 0.24583333 0.25 0.25416667 0.25833333 0.2625 0.26666667 0.27083333 0.275 0.27916667 0.28333333 0.2875 0.29166667 0.29583333 0.3 0.30416667 0.30833333 0.3125 0.31666667 0.32083333 0.325 0.32916667 0.33333333 0.3375 0.34166667 0.34583333 0.35 0.35416667 0.35833333 0.3625 0.36666667 0.37083333 0.375 0.37916667 0.38333333 0.3875 0.39166667 0.39583333 0.4 0.40416667 0.40833333 0.4125 0.41666667 0.42083333 0.425 0.42916667 0.43333333 0.4375 0.44166667 0.44583333 0.45 0.45416667 0.45833333 0.4625 0.46666667 0.47083333 0.475 0.47916667 0.48333333 0.4875 0.49166667 0.49583333 0.5 0.50416667 0.50833333 0.5125 0.51666667 0.52083333 0.525 0.52916667 0.53333333 0.5375 0.54166667 0.54583333 0.55 0.55416667 0.55833333 0.5625 0.56666667 0.57083333 0.575 0.57916667 0.58333333 0.5875 0.59166667 0.59583333 0.6 0.60416667 0.60833333 0.6125 0.61666667 0.62083333 0.625 0.62916667 0.63333333 0.6375 0.64166667 0.64583333 0.65 0.65416667 0.65833333 0.6625 0.66666667 0.67083333 0.675 0.67916667 0.68333333 0.6875 0.69166667 0.69583333 0.7 0.70416667 0.70833333 0.7125 0.71666667 0.72083333 0.725 0.72916667 0.73333333 0.7375 0.74166667 0.74583333 0.75 0.75416667 0.75833333 0.7625 0.76666667 0.77083333 0.775 0.77916667 0.78333333 0.7875 0.79166667 0.79583333 0.8 0.80416667 0.80833333 0.8125 0.81666667 0.82083333 0.825 0.82916667 0.83333333 0.8375 0.84166667 0.84583333 0.85 0.85416667 0.85833333 0.8625 0.86666667 0.87083333 0.875 0.87916667 0.88333333 0.8875 0.89166667 0.89583333 0.9 0.90416667 0.90833333 0.9125 0.91666667 0.92083333 0.925 0.92916667 0.93333333 0.9375 0.94166667 0.94583333 0.95 0.95416667 0.95833333 0.9625 0.96666667 0.97083333 0.975 0.97916667 0.98333333 0.9875 0.99166667 0.99583333 1 1 1 1 1 1
  arc A17 (-25.363, -5.3246) -> (-24.7898, -6.1136) centre (0, 12.5) ccw
  spline S17 degree 5 poles (-24.7898, -6.1136) (-24.7872, -6.1128) (-24.782, -6.1113) (-24.7743, -6.109) (-24.7639, -6.1059) (-24.751, -6.1021) (-24.7382, -6.0982) (-24.7253, -6.0943) (-24.7125, -6.0905) (-24.6998, -6.0866) (-24.6871, -6.0827) (-24.6744, -6.0788) (-24.6617, -6.0749) (-24.6491, -6.071) (-24.6365, -6.0671) (-24.624, -6.0632) (-24.6115, -6.0593) (-24.599, -6.0553) (-24.5866, -6.0514) (-24.5742, -6.0475) (-24.5618, -6.0435) (-24.5495, -6.0395) (-24.5372, -6.0356) (-24.5249, -6.0316) (-24.5127, -6.0277) (-24.5005, -6.0237) (-24.4884, -6.0197) (-24.4762, -6.0157) (-24.4642, -6.0117) (-24.4521, -6.0077) (-24.4401, -6.0037) (-24.4281, -5.9997) (-24.4162, -5.9957) (-24.4043, -5.9917) (-24.3925, -5.9877) (-24.3806, -5.9836) (-24.3689, -5.9796) (-24.3571, -5.9756) (-24.3454, -5.9715) (-24.3337, -5.9675) (-24.3221, -5.9634) (-24.3105, -5.9594) (-24.299, -5.9553) (-24.2874, -5.9513) (-24.276, -5.9472) (-24.2645, -5.9431) (-24.2531, -5.9391) (-24.2417, -5.935) (-24.2304, -5.9309) (-24.2191, -5.9269) (-24.2079, -5.9228) (-24.1967, -5.9187) (-24.1855, -5.9146) (-24.1744, -5.9105) (-24.1633, -5.9064) (-24.1522, -5.9023) (-24.1412, -5.8982) (-24.1302, -5.8941) (-24.1193, -5.89) (-24.1084, -5.8859) (-24.0975, -5.8818) (-24.0867, -5.8777) (-24.0759, -5.8736) (-24.0652, -5.8695) (-24.0545, -5.8654) (-24.0438, -5.8613) (-24.0332, -5.8572) (-24.0226, -5.8531) (-24.0121, -5.849) (-24.0016, -5.8449) (-23.9911, -5.8408) (-23.9807, -5.8366) (-23.9703, -5.8325) (-23.96, -5.8284) (-23.9497, -5.8243) (-23.9395, -5.8202) (-23.9292, -5.8161) (-23.9191, -5.812) (-23.909, -5.8079) (-23.8989, -5.8038) (-23.8888, -5.7996) (-23.8788, -5.7955) (-23.8689, -5.7914) (-23.859, -5.7873) (-23.8491, -5.7832) (-23.8393, -5.7791) (-23.8295, -5.775) (-23.8197, -5.7709) (-23.81, -5.7668) (-23.8004, -5.7627) (-23.7907, -5.7587) (-23.7812, -5.7546) (-23.7716, -5.7505) (-23.7622, -5.7464) (-23.7527, -5.7423) (-23.7433, -5.7383) (-23.734, -5.7342) (-23.7247, -5.7301) (-23.7154, -5.726) (-23.7062, -5.722) (-23.697, -5.7179) (-23.6879, -5.7139) (-23.6788, -5.7098) (-23.6697, -5.7058) (-23.6607, -5.7018) (-23.6518, -5.6977) (-23.6429, -5.6937) (-23.634, -5.6897) (-23.6252, -5.6857) (-23.6165, -5.6816) (-23.6077, -5.6776) (-23.5991, -5.6736) (-23.5904, -5.6696) (-23.5818, -5.6657) (-23.5733, -5.6617) (-23.5648, -5.6577) (-23.5564, -5.6537) (-23.548, -5.6498) (-23.5396, -5.6458) (-23.5313, -5.6419) (-23.5231, -5.6379) (-23.5149, -5.634) (-23.5067, -5.6301) (-23.4986, -5.6262) (-23.4905, -5.6223) (-23.4825, -5.6184) (-23.4746, -5.6145) (-23.4666, -5.6106) (-23.4588, -5.6068) (-23.451, -5.6029) (-23.4432, -5.5991) (-23.4355, -5.5952) (-23.4278, -5.5914) (-23.4202, -5.5876) (-23.4126, -5.5838) (-23.4051, -5.58) (-23.3976, -5.5762) (-23.3902, -5.5724) (-23.3828, -5.5687) (-23.3755, -5.5649) (-23.3683, -5.5612) (-23.361, -5.5575) (-23.3539, -5.5538) (-23.3468, -5.5501) (-23.3397, -5.5464) (-23.3327, -5.5427) (-23.3257, -5.539) (-23.3188, -5.5354) (-23.312, -5.5318) (-23.3052, -5.5282) (-23.2984, -5.5246) (-23.2918, -5.521) (-23.2851, -5.5174) (-23.2785, -5.5139) (-23.272, -5.5103) (-23.2655, -5.5068) (-23.2591, -5.5033) (-23.2527, -5.4998) (-23.2464, -5.4963) (-23.2402, -5.4929) (-23.234, -5.4895) (-23.2278, -5.486) (-23.2217, -5.4826) (-23.2157, -5.4793) (-23.2097, -5.4759) (-23.2038, -5.4726) (-23.1979, -5.4692) (-23.1921, -5.4659) (-23.1864, -5.4627) (-23.1807, -5.4594) (-23.1751, -5.4562) (-23.1695, -5.4529) (-23.164, -5.4497) (-23.1585, -5.4466) (-23.1531, -5.4434) (-23.1478, -5.4403) (-23.1425, -5.4372) (-23.1373, -5.4341) (-23.1321, -5.431) (-23.127, -5.428) (-23.122, -5.425) (-23.117, -5.422) (-23.1121, -5.4191) (-23.1072, -5.4161) (-23.1024, -5.4132) (-23.0977, -5.4103) (-23.093, -5.4075) (-23.0884, -5.4047) (-23.0839, -5.4019) (-23.0794, -5.3991) (-23.075, -5.3964) (-23.0706, -5.3937) (-23.0664, -5.391) (-23.0621, -5.3883) (-23.058, -5.3857) (-23.0539, -5.3831) (-23.0499, -5.3806) (-23.0459, -5.3781) (-23.042, -5.3756) (-23.0382, -5.3731) (-23.0344, -5.3707) (-23.0308, -5.3683) (-23.0271, -5.366) (-23.0236, -5.3637) (-23.0201, -5.3614) (-23.0167, -5.3592) (-23.0134, -5.357) (-23.0101, -5.3548) (-23.0069, -5.3527) (-23.0038, -5.3506) (-23.0007, -5.3485) (-22.9978, -5.3465) (-22.9948, -5.3446) (-22.992, -5.3427) (-22.9893, -5.3408) (-22.9866, -5.3389) (-22.984, -5.3372) (-22.9814, -5.3354) (-22.979, -5.3337) (-22.9766, -5.3321) (-22.9743, -5.3305) (-22.9721, -5.3289) (-22.9699, -5.3274) (-22.9679, -5.326) (-22.9659, -5.3246) (-22.964, -5.3232) (-22.9622, -5.3219) (-22.9604, -5.3207) (-22.9588, -5.3195) (-22.9572, -5.3183) (-22.9557, -5.3172) (-22.9543, -5.3162) (-22.953, -5.3153) (-22.9518, -5.3144) (-22.9506, -5.3135) (-22.9496, -5.3127) (-22.9486, -5.312) (-22.9477, -5.3114) (-22.9469, -5.3108) (-22.9463, -5.3103) (-22.9457, -5.3098) (-22.9453, -5.3095) (-22.945, -5.3093) (-22.9448, -5.3092) (-22.9448, -5.3091) knots -1 -1 -1 -1 -1 -1 -0.99583333 -0.99166667 -0.9875 -0.98333333 -0.97916667 -0.975 -0.97083333 -0.96666667 -0.9625 -0.95833333 -0.95416667 -0.95 -0.94583333 -0.94166667 -0.9375 -0.93333333 -0.92916667 -0.925 -0.92083333 -0.91666667 -0.9125 -0.90833333 -0.90416667 -0.9 -0.89583333 -0.89166667 -0.8875 -0.88333333 -0.87916667 -0.875 -0.87083333 -0.86666667 -0.8625 -0.85833333 -0.85416667 -0.85 -0.84583333 -0.84166667 -0.8375 -0.83333333 -0.82916667 -0.825 -0.82083333 -0.81666667 -0.8125 -0.80833333 -0.80416667 -0.8 -0.79583333 -0.79166667 -0.7875 -0.78333333 -0.77916667 -0.775 -0.77083333 -0.76666667 -0.7625 -0.75833333 -0.75416667 -0.75 -0.74583333 -0.74166667 -0.7375 -0.73333333 -0.72916667 -0.725 -0.72083333 -0.71666667 -0.7125 -0.70833333 -0.70416667 -0.7 -0.69583333 -0.69166667 -0.6875 -0.68333333 -0.67916667 -0.675 -0.67083333 -0.66666667 -0.6625 -0.65833333 -0.65416667 -0.65 -0.64583333 -0.64166667 -0.6375 -0.63333333 -0.62916667 -0.625 -0.62083333 -0.61666667 -0.6125 -0.60833333 -0.60416667 -0.6 -0.59583333 -0.59166667 -0.5875 -0.58333333 -0.57916667 -0.575 -0.57083333 -0.56666667 -0.5625 -0.55833333 -0.55416667 -0.55 -0.54583333 -0.54166667 -0.5375 -0.53333333 -0.52916667 -0.525 -0.52083333 -0.51666667 -0.5125 -0.50833333 -0.50416667 -0.5 -0.49583333 -0.49166667 -0.4875 -0.48333333 -0.47916667 -0.475 -0.47083333 -0.46666667 -0.4625 -0.45833333 -0.45416667 -0.45 -0.44583333 -0.44166667 -0.4375 -0.43333333 -0.42916667 -0.425 -0.42083333 -0.41666667 -0.4125 -0.40833333 -0.40416667 -0.4 -0.39583333 -0.39166667 -0.3875 -0.38333333 -0.37916667 -0.375 -0.37083333 -0.36666667 -0.3625 -0.35833333 -0.35416667 -0.35 -0.34583333 -0.34166667 -0.3375 -0.33333333 -0.32916667 -0.325 -0.32083333 -0.31666667 -0.3125 -0.30833333 -0.30416667 -0.3 -0.29583333 -0.29166667 -0.2875 -0.28333333 -0.27916667 -0.275 -0.27083333 -0.26666667 -0.2625 -0.25833333 -0.25416667 -0.25 -0.24583333 -0.24166667 -0.2375 -0.23333333 -0.22916667 -0.225 -0.22083333 -0.21666667 -0.2125 -0.20833333 -0.20416667 -0.2 -0.19583333 -0.19166667 -0.1875 -0.18333333 -0.17916667 -0.175 -0.17083333 -0.16666667 -0.1625 -0.15833333 -0.15416667 -0.15 -0.14583333 -0.14166667 -0.1375 -0.13333333 -0.12916667 -0.125 -0.12083333 -0.11666667 -0.1125 -0.10833333 -0.10416667 -0.1 -0.09583333 -0.09166667 -0.0875 -0.08333333 -0.07916667 -0.075 -0.07083333 -0.06666667 -0.0625 -0.05833333 -0.05416667 -0.05 -0.04583333 -0.04166667 -0.0375 -0.03333333 -0.02916667 -0.025 -0.02083333 -0.01666667 -0.0125 -0.00833333 -0.00416667 0 0 0 0 0 0
  line L43 (-22.9448, -5.3091) -> (-22.9441, -5.3086)
  line L44 (-22.9441, -5.3086) -> (-22.7115, -5.1281)
  arc A18 (-22.7115, -5.1281) -> (-21.9649, -6.0501) centre (0, 12.5) ccw
  line L45 (-21.9649, -6.0501) -> (-22.1898, -6.2401)
  line L46 (-22.1898, -6.2401) -> (-22.1904, -6.2406)